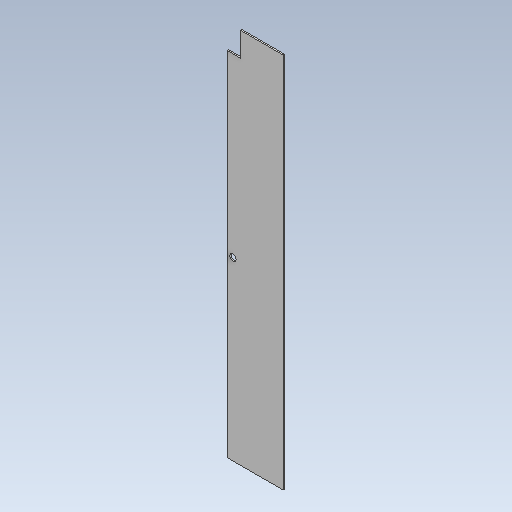
# Autodesk Inventor part: Part15
Saved by Autodesk Inventor 2020.2 (Build 242310000, 310)
## iProperties
Created: 2022-11-15
Part Number: Part15
Material: 一般
Document SubType Name: Modeling
Designer: Administrator
Density: 1 g/cm^3
Appearance: 既定
Author: Administrator
Autodesk Inventor part; units mm, degrees
ref_plane "YZ Plane" through (0, 0, 0) normal (1, 0, 0) x (0, 1, 0)
ref_plane "XZ Plane" through (0, 0, 0) normal (0, 1, 0) x (-1, 0, 0)
ref_plane "XY Plane" through (0, 0, 0) normal (0, 0, 1) x (1, 0, 0)
sketch "スケッチ1" plane through (0, 0, 0) normal (0, 0, 1) x (1, 0, 0)
  circle A0 centre (9, 227.5) radius 2.75 projected
  line L0 (14, 222) -> (14, 233) projected
  line L1 (0, 233) -> (14, 233) projected
  line L2 (0, 222) -> (0, 233) projected
  line L3 (14, 222) -> (0, 222) projected
  circle A1 centre (9, 273) radius 2.75 projected
  line L4 (14, 267.5) -> (14, 278.5) projected
  line L5 (0, 278.5) -> (14, 278.5) projected
  line L6 (0, 267.5) -> (0, 278.5) projected
  line L7 (14, 267.5) -> (0, 267.5) projected
  circle A2 centre (-23, 227.5) radius 2.75 projected
  line L8 (-14, 222) -> (-14, 233) projected
  line L9 (-28, 233) -> (-14, 233) projected
  line L10 (-28, 222) -> (-28, 233) projected
  line L11 (-14, 222) -> (-28, 222) projected
  circle A3 centre (-23, 273) radius 2.75 projected
  line L12 (-14, 267.5) -> (-14, 278.5) projected
  line L13 (-28, 278.5) -> (-14, 278.5) projected
  line L14 (-28, 267.5) -> (-28, 278.5) projected
  line L15 (-14, 267.5) -> (-28, 267.5) projected
  line L16 (14, 233) -> (-28, 233)
  line L17 (-28, 233) -> (-28, 267.5)
  line L18 (-28, 267.5) -> (14, 267.5)
  line L19 (14, 267.5) -> (14, 233)
  line L20 (-7, 233) -> (33, 233)
  line L21 (-7, 267.5) -> (33, 267.5)
  line L22 (33, 267.5) -> (33, 233)
  line L23 (33, 233) -> (-47, 233)
  line L24 (-47, 233) -> (-47, -272.0187)
  line L25 (-47, -272.0187) -> (33, -272.0187)
  line L26 (33, -272.0187) -> (33, 233)
  line L27 (33, 233) -> (33, -19.5093)
  line L28 (-47, 233) -> (-47, -19.5093)
  line L29 (33, -19.5093) -> (-47, -19.5093)
  circle A4 centre (25, 26.7655) radius 4.5 projected
  circle A5 centre (-39, 26.7655) radius 4.5 projected
  circle A6 centre (25, -19.5093) radius 4.5662
  circle A7 centre (-39, -19.5093) radius 4.5662
  point P0 (0, 0)
  point P1 (14, -5.5)
  point P2 (0, 5.5)
  point P3 (-14, 5.5)
  point P4 (-28, -33.5187)
  point P5 (-14, -44.5187)
  point P6 (0, -44.5187)
  point P7 (14, 267.5)
  point P8 (-28, -43.5187)
  point P9 (-28, 233)
  point P10 (-34.4338, -19.5093)
  point P11 (-43.5662, -19.5093)
  point P12 (-43.4328, -19.5093)
  point P13 (-43.5, -18.7345)
  point P14 (-34.5, -18.7345)
  point P15 (-34.5672, -19.5093)
  point P16 (29.5662, -19.5093)
  point P17 (20.4338, -19.5093)
  point P18 (20.5672, -19.5093)
  point P19 (20.5, -18.7345)
  point P20 (29.5, -18.7345)
  point P21 (29.4328, -19.5093)
  point P22 (14, 267.5)
  point P23 (14, 267.5)
  point P24 (0, 267.5)
  point P25 (0, 233)
  dimension "d2" = 40
  dimension "d3" = 80
  constraints: 28 end point, 4 horizontal, 4 midpoint, 4 parallel, 4 perpendicular, 2 centre point, 2 point on line
  measures "d2" distance of L20.start L20.end
  measures "d3" distance of L25.end L24.end
extrude "押し出し1" add sketch "スケッチ1" along normal blind 2 contours A0 | L3 L2 L1 L0 | L0 L20 L26 L29 A6 A7 L24 L23 L10 L11 L8 L16 L2 L3 | L1 L16 L9 L17 L15 L18 L7 L19 | L19 L21 L22 L20 | L26 L25 L24 L29 A7 A6 | L8 L11 L10 L9 | A2 | A4 | A5
